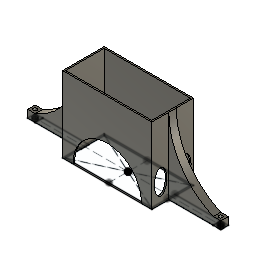
PSU mount (Autodesk Fusion 360 design; units mm, degrees)
Autodesk Fusion 360 part; units mm, degrees
sketch "Sketch1" plane through (0, 0, 0) normal (0, 0, 1) x (1, 0, 0)
  line L0 (0, 0) -> (-122.75, 0) construction
  line L1 (0, 0) -> (0, 25.25) construction
  line L2 (0, 0) -> (122.75, 0) construction
  line L3 (0, 0) -> (0, -25.25) construction
  circle A0 centre (-122.75, 0) radius 2.5
  circle A1 centre (122.75, 0) radius 2.5
  line L4 (-57, 25.5) -> (57, 25.5)
  line L5 (57, 25.5) -> (57, -25.5)
  line L6 (57, -25.5) -> (-57, -25.5)
  line L7 (-57, -25.5) -> (-57, 25.5)
  line L8 (-57, 25.5) -> (57, -25.5) construction
  line L9 (57, 25.5) -> (-57, -25.5) construction
  line L10 (-117.75, 5) -> (-127.75, 5)
  line L11 (-127.75, 5) -> (-127.75, -5)
  line L12 (-127.75, -5) -> (-117.75, -5)
  line L13 (-117.75, -5) -> (-117.75, 5)
  line L14 (-117.75, 5) -> (-127.75, -5) construction
  line L15 (-127.75, 5) -> (-117.75, -5) construction
  line L16 (-117.75, 5) -> (-57, 5)
  line L17 (-57, 5) -> (-57, -5)
  line L18 (-57, -5) -> (-117.75, -5)
  line L19 (-117.75, -5) -> (-117.75, 5)
  line L20 (117.75, -5) -> (117.75, 5)
  line L21 (127.75, 5) -> (127.75, -5)
  line L22 (117.75, 5) -> (127.75, -5) construction
  line L23 (117.75, -5) -> (117.75, 5)
  line L24 (127.75, 5) -> (117.75, -5) construction
  line L25 (127.75, -5) -> (117.75, -5)
  line L26 (117.75, 5) -> (127.75, 5)
  circle A2 centre (122.75, 0) radius 2.5
  line L27 (117.75, 5) -> (57, 5)
  line L28 (57, -5) -> (117.75, -5)
  line L29 (59, 27.5) -> (-59, 27.5)
  line L30 (-59, 27.5) -> (-59, -27.5)
  line L31 (-59, -27.5) -> (59, -27.5)
  line L32 (59, -27.5) -> (59, 27.5)
  line L33 (59, 27.5) -> (-59, -27.5) construction
  line L34 (-59, 27.5) -> (59, -27.5) construction
  point P0 (-122.75, 0)
  point P1 (122.75, 0)
  point P2 (122.75, 0)
  dimension "d1" = 122.75
  dimension "d2" = 25.25
  dimension "d3" = 5
  dimension "d4" = 114
  dimension "d5" = 51
  dimension "d6" = 10
  dimension "d7" = 10
  dimension "d8" = 10
  dimension "d19" = 118
  dimension "d20" = 55
  constraint coincident L0.start L1.start
  constraint horizontal L0
  constraint perpendicular L0 L1
  constraint symmetric L0.start L1 L2.start
  constraint symmetric P0 L1 P1
  constraint symmetric L0 L1.start L2.start
  constraint symmetric L0 L1.end L3.end
  constraint coincident P0 L0.end
  constraint symmetric L1 A0 A1
  constraint horizontal L4
  constraint perpendicular L4 L5
  constraint parallel L4 L6
  constraint parallel L5 L7
  constraint coincident L8 L0.start
  constraint coincident L9 L0.start
  constraint horizontal L10
  constraint perpendicular L10 L11
  constraint parallel L10 L12
  constraint parallel L11 L13
  constraint coincident L14 P0
  constraint coincident L15 P0
  constraint horizontal L16
  constraint vertical L17
  constraint horizontal L18
  constraint vertical L19
  constraint coincident L7 L17.end
  constraint symmetric L1 A0 A2
  constraint symmetric L1 L10.start L20.end
  constraint symmetric L1 L10.end L21.start
  constraint symmetric L1 L11.end L21.end
  constraint symmetric L1 L12.end L20.start
  constraint symmetric L1 P0 P2
  constraint symmetric L1 L16.end L27.end
  constraint symmetric L1 L17.end L28.start
  constraint horizontal L29
  constraint perpendicular L29 L30
  constraint parallel L29 L31
  constraint parallel L30 L32
  constraint coincident L33 L0.start
  constraint coincident L34 L0.start
  measures "d1" distance of L0.start P0
  measures "d2" distance of L0.start L1.end
  measures "d3" diameter of A0
  measures "d4" distance of L5.end L6.end
  measures "d5" distance of L4.end L5.end
  measures "d6" distance of L11.end L12.end
  measures "d7" distance of L10.end L11.end
  measures "d8" distance of L10.start L12.end
  measures "d19" distance of L30.end L31.end
  measures "d20" distance of L29.end L30.end
extrude "Extrude2" add sketch "Sketch1" along normal blind 10 contours L10 L11 L12 L13 L19 | L20 L21 L23 L25 L26 makes body 1 at (125.2469, -0.1246, 6.6667) makes body 2 at (-120.2531, -0.1246, 6.6667)
sketch "Sketch2" plane through (0, 5, 0) normal (0, 1, 0) x (-1, 0, 0)
  line L0 (117.75, 0) -> (127.75, 0)
  line L1 (127.75, 0) -> (127.75, 10)
  line L2 (127.75, 10) -> (117.75, 10)
  arc A0 (57, 100) -> (117.75, 10) centre (154.0417, 100) ccw
  line L3 (117.75, 10) -> (117.75, 0)
  constraint coincident L2.end A0.end
sketch "Sketch3" plane through (0, 5, 0) normal (0, 1, 0) x (-1, 0, 0)
  line L0 (-127.75, 0) -> (-117.75, 0)
  line L1 (-117.75, 10) -> (-127.75, 10)
  line L2 (-127.75, 10) -> (-127.75, 0)
  arc A0 (-117.75, 10) -> (-57, 100) centre (-154.0417, 100) ccw
  line L3 (-117.75, 0) -> (-117.75, 10)
  constraint coincident L1.start A0.start
extrude "Extrude7" add sketch "Sketch1" along normal blind 100 separate body contours L4 L5 L7 L16 L27 L29 L30 L32 | L7 L16 L17 L18 L30 | L5 L27 L28 L32 | L5 L6 L7 L18 L28 L30 L31 L32 makes body 3
extrude "Extrude8" add sketch "Sketch1" along normal blind 100 contours L13 L16 L18 L19 L30 | L20 L23 L27 L28 L32 bodies 1 2 3
sketch "Sketch4" plane through (0, -5, 0) normal (0, -1, 0) x (1, 0, 0)
  line L0 (-127.75, 0) -> (-59, 0)
  line L1 (-59, 0) -> (-59, 100)
  line L2 (-59, 100) -> (-117.75, 100)
  line L3 (-117.75, 100) -> (-117.75, 10)
  line L4 (-117.75, 10) -> (-127.75, 10)
  line L5 (-127.75, 10) -> (-127.75, 0)
  arc A0 (-117.75, 10) -> (-59, 100) centre (-154.7515, 98.3291) ccw
  constraint coincident L3.end L4.start
  constraint coincident L1.end L2.start
sketch "Sketch5" plane through (0, -5, 0) normal (0, -1, 0) x (1, 0, 0)
  line L0 (59, 0) -> (127.75, 0)
  line L1 (127.75, 0) -> (127.75, 10)
  line L2 (127.75, 10) -> (117.75, 10)
  line L3 (117.75, 10) -> (117.75, 100)
  line L4 (117.75, 100) -> (59, 100)
  line L5 (59, 100) -> (59, 0)
  arc A0 (59, 100) -> (117.75, 10) centre (157.3112, 100) ccw
  constraint tangent L5 A0
  constraint coincident L2.end L3.start
  constraint coincident L4.end L5.start
extrude "Extrude9" cut sketch "Sketch5" sketch "Sketch4" against normal blind 35 contours L3 L4 A0 of sketch 2 contours L1 L2 L3 A0 bodies 1
sketch "Sketch6" plane through (0, -27.5, 0) normal (0, -1, 0) x (1, 0, 0)
  line L0 (-59, 0) -> (59, 0)
  line L1 (59, 0) -> (59, 100)
  line L2 (59, 100) -> (-59, 100)
  line L3 (-59, 100) -> (-59, 0)
  line L4 (-45, 0) -> (45, 0) construction
  line L5 (45, 0) -> (45, 37.4909) construction
  line L6 (45, 37.4909) -> (-45, 37.4909) construction
  line L7 (-45, 37.4909) -> (-45, 0) construction
  line L8 (-45, 0) -> (45, 37.4909) construction
  line L9 (45, 0) -> (-45, 37.4909) construction
  arc A0 (45, 0) -> (-45, 0) centre (0, 1.4121) ccw
  point P0 (0, 18.7455)
  dimension "d29" = 90
  constraint horizontal L4
  constraint perpendicular L4 L5
  constraint parallel L4 L6
  constraint parallel L5 L7
  constraint coincident L8 P0
  constraint coincident L9 P0
  measures "d29" distance of L5.end L6.end
extrude "Extrude10" cut sketch "Sketch6" against normal blind 95 contours L0 A0 bodies 1
sketch "Sketch7" plane through (-59, 0, 0) normal (-1, 0, 0) x (0, -1, 0)
  line L0 (-27.5, 100) -> (-27.5, 0)
  line L1 (-27.5, 0) -> (-5, 0)
  line L2 (-5, 0) -> (-5, 96.6583)
  line L3 (-5, 96.6583) -> (5, 96.6583)
  line L4 (5, 96.6583) -> (5, 0)
  line L5 (5, 0) -> (27.5, 0)
  line L6 (27.5, 0) -> (27.5, 100)
  line L7 (27.5, 100) -> (-27.5, 100)
  ellipse E0 centre (-16.1457, 25.858) end of major axis (-16.1457, 9.4792) minor radius 8.2129
  line L8 (-16.1457, 42.2368) -> (-16.1457, 9.4792) construction
  line L9 (-24.3586, 25.858) -> (-7.9328, 25.858) construction
  ellipse E1 centre (15.8543, 25.858) end of major axis (15.8543, 9.4792) minor radius 8.2129
  line L10 (15.8543, 42.2368) -> (15.8543, 9.4792) construction
  line L11 (7.6414, 25.858) -> (24.0672, 25.858) construction
  point P0 (-16.1457, 25.858)
  constraint coincident E0 L8.start
  constraint coincident E0 L8.end
  constraint coincident E0 L9.start
  constraint coincident E0 L9.end
  constraint parallel L2 L8
  constraint coincident E1 L10.start
  constraint coincident E1 L10.end
  constraint coincident E1 L11.start
  constraint coincident E1 L11.end
extrude "Extrude11" cut sketch "Sketch7" against normal blind 145 contours E0 | E1 bodies 1
equation "d1 = ( 245.5 / 2 ) * 1 mm"
